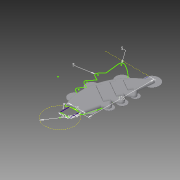
# Autodesk Inventor part: EarWing
Saved by Autodesk Inventor 2014 SP1 (Build 180222100, 222)
## iProperties
Created: 2015-03-17
Part Number: EarWing
Material: Generic
Document SubType Name: Modeling
Designer: Erin
Density: 1 g/cm^3
Appearance: Default
Author: Erin
Autodesk Inventor part; units mm, degrees
ref_plane "YZ Plane" through (0, 0, 0) normal (1, 0, 0) x (0, 1, 0)
ref_plane "XZ Plane" through (0, 0, 0) normal (0, 1, 0) x (-1, 0, 0)
sketch "Sketch1" plane through (0, 0, 0) normal (0, 0, 1) x (1, 0, 0)
  line L0 (-10, -4.740173) -> (10, -4.740173)
  line L1 (10, -4.740173) -> (10, -24.740173)
  line L2 (10, -24.740173) -> (-10, -24.740173)
  line L3 (-10, -24.740173) -> (-10, -4.740173)
  line L4 (-17.5, -4.740173) -> (17.5, -4.740173)
  line L5 (17.5, -4.740173) -> (17.5, 130.259827) construction
  line L6 (17.5, 130.259827) -> (-71.879841, 130.259827) construction
  arc A0 (17.5, -4.740173) -> (-28.622314, 126.472101) centre (-75.017769, 36.45133) ccw
  line L7 (-35.882424, 121.476257) -> (-32.663792, 92.468063)
  line L8 (-32.663792, 92.468063) -> (-40.677059, 83.337371)
  line L9 (-39.242537, 75.611926) -> (-29.283469, 70.385393)
  line L10 (-29.283469, 70.385393) -> (-38.911262, 59.415034)
  line L11 (-37.47674, 51.689589) -> (-26.78782, 46.080029)
  line L12 (-26.78782, 46.080029) -> (-34.350121, 37.463189)
  arc A1 (-28.622314, 126.472101) -> (-35.882424, 121.476257) centre (-30.912921, 122.027653) ccw
  line L13 (-32.915599, 29.737744) -> (-24.548066, 25.346451)
  line L14 (-24.548066, 25.346451) -> (-17.5, -4.740173)
  arc A2 (-40.677059, 83.337371) -> (-39.242537, 75.611926) centre (-36.919057, 80.039278) ccw
  arc A3 (-38.911262, 59.415034) -> (-37.47674, 51.689589) centre (-35.15326, 56.116941) ccw
  arc A4 (-34.350121, 37.463189) -> (-32.915599, 29.737744) centre (-30.592119, 34.165096) ccw
  circle A5 centre (0, -34.740173) radius 30 construction
  arc A6 (15.764218, -8.047675) -> (-16.074353, -8.233283) centre (0, -34.740173) ccw
  line L15 (-17.5, -4.740173) -> (-16.074353, -8.233283)
  line L16 (17.5, -4.740173) -> (15.764218, -8.047675)
  line L17 (-10, -4.740173) -> (10, -4.740173)
  line L18 (10, -4.740173) -> (10, -1.45931)
  line L19 (10, -1.45931) -> (-10, -1.45931)
  line L20 (-10, -1.45931) -> (-10, -4.740173)
  point P0 (0, 0)
  point P1 (0, -4.740173)
  point P2 (-36.857014, 130.259827)
  point P3 (0, -4.740173)
  dimension "d0" = 20
  dimension "d1" = 20
  dimension "d2" = 35
  dimension "d3" = 135
  dimension "d4" = 5
  dimension "d5" = 5
  dimension "d6" = 60
  dimension "d7" = 1
  constraints: 42 end point, 13 point on circle, 9 tangent, 8 parallel, 7 centre point, 6 perpendicular, 2 equal radius, 2 horizontal, 2 midpoint, 2 point on line, 2 vertical alignment, 1 collinear
  measures "d0" distance of L1.end L2.end
  measures "d1" distance of L0.end L1.end
  measures "d2" distance of L4.start L4.end
  measures "d3" distance of L4.end L5.end
  measures "d4" radius of A1
  measures "d5" radius of A2
  measures "d6" diameter of A5
  measures "d7" radial gap between concentric circles of A5 A6
extrude "Extrusion1" add sketch "Sketch1" along normal blind 3 contours L20 L19 L18 L0 A6 | L0 A6 L3 | L3 A6 L15 L4 | L4 L14 L13 A4 L12 L11 A3 L10 L9 A2 L8 L7 A1 A0 L18 L19 L20 | L0 L1 A6 | L4 L16 A6 L1
fillet "Fillet1" radius 5 13 edges at (-33.7473, 126.1467, 3) (-34.2731, 106.9722, 3) (20.5248, 70.0354, 3) (-41.835, 79.1264, 3) (-34.263, 72.9987, 3) (-36.6704, 87.9027, 3) (-40.0692, 55.2041, 3) (-32.1323, 48.8848, 3) (-34.0974, 64.9002, 3) (-35.5081, 33.2523, 3) (-28.7318, 27.5421, 3) (-30.569, 41.7716, 3) (-21.024, 10.3031, 3)
ref_plane "Work Plane1" through (0, 0, 3) normal (0, 0, 1) x (1, 0, 0)
sketch "Sketch2" plane through (0, 0, 3) normal (0, 0, 1) x (1, 0, 0)
  arc A0 (17.5, -4.740173) -> (-28.622314, 126.472101) centre (-75.017769, 36.45133) ccw
  arc A1 (17.5, -4.740173) -> (-28.622314, 126.472101) centre (-75.017769, 36.45133) ccw
  line L0 (-35.882424, 121.476257) -> (-32.663792, 92.468063)
  line L1 (-32.663792, 92.468063) -> (-40.677059, 83.337371)
  arc A2 (-40.677059, 83.337371) -> (-39.242537, 75.611926) centre (-36.919057, 80.039278) ccw
  line L2 (-39.242537, 75.611926) -> (-29.283469, 70.385393)
  line L3 (-29.283469, 70.385393) -> (-38.911262, 59.415034)
  arc A3 (-38.911262, 59.415034) -> (-37.47674, 51.689589) centre (-35.15326, 56.116941) ccw
  line L4 (-37.47674, 51.689589) -> (-26.78782, 46.080029)
  line L5 (-26.78782, 46.080029) -> (-34.350121, 37.463189)
  arc A4 (-34.350121, 37.463189) -> (-32.915599, 29.737744) centre (-30.592119, 34.165096) ccw
  line L6 (-32.915599, 29.737744) -> (-24.548066, 25.346451)
  line L7 (-24.548066, 25.346451) -> (-17.5, -4.740173)
  line L8 (-17.5, -4.740173) -> (-17.5, -4.740173)
  arc A5 (-10, -5.397371) -> (-16.074353, -8.233283) centre (0, -34.740173) ccw
  arc A6 (15.764218, -8.047675) -> (-16.074353, -8.233283) centre (0, -34.740173) ccw
  line L9 (17.5, -4.740173) -> (15.764218, -8.047675)
  line L10 (-28.692137, 88.355038) -> (-5.168136, 101.909269)
  line L11 (-5.168136, 101.909269) -> (-0.503674, 93.813876)
  line L12 (-0.503674, 93.813876) -> (-24.027675, 80.259646)
  line L13 (-24.027675, 80.259646) -> (-28.692137, 88.355038)
  line L14 (-28.000372, 65.795929) -> (5.455455, 85.072752)
  line L15 (5.455455, 85.072752) -> (10.119917, 76.977359)
  line L16 (10.119917, 76.977359) -> (-23.33591, 57.700537)
  line L17 (-23.33591, 57.700537) -> (-28.000372, 65.795929)
  line L18 (-23.904487, 43.113193) -> (13.330015, 64.567241)
  line L19 (13.330015, 64.567241) -> (17.994477, 56.471849)
  line L20 (17.994477, 56.471849) -> (-19.240025, 35.017801)
  line L21 (-19.240025, 35.017801) -> (-23.904487, 43.113193)
  point P0 (0, 0)
  point P1 (-16.074353, -8.233283)
  constraints: 24 end point, 6 parallel, 3 perpendicular, 2 other
extrude "Extrusion3" add sketch "Sketch2" along normal blind 1.5
fillet "Fillet2" radius 5 6 edges at (-26.3599, 84.3073, 4.5) (-25.6681, 61.7482, 4.5) (-21.5723, 39.0655, 4.5) (7.7877, 81.0251, 4.5) (-2.8359, 97.8616, 4.5) (15.6622, 60.5195, 4.5)
sketch "Sketch3" plane through (0, 0, 0) normal (0, 0, 1) x (1, 0, 0)
  circle A0 centre (-30.567755, 123.082332) radius 14.903634
  circle A1 centre (3.412533, 95.957719) radius 12.733671
  circle A2 centre (22.191113, 52.737181) radius 11.866888
  circle A3 centre (20.70075, 16.372315) radius 12.43717
  circle A4 centre (-15.988631, 8.920494) radius 11.808181
  circle A5 centre (-32.356191, 33.660528) radius 8.690238
  circle A6 centre (-37.125354, 56.015978) radius 8.966984
  circle A7 centre (-38.91379, 81.054085) radius 7.772792
  point P0 (0, 0)
  constraints: 8 centre point
extrude "Extrusion4" add sketch "Sketch3" along normal blind 0.3
fillet "Fillet3" radius 3 3 edges at (14.3155, -7.2435, 2.1718) (-14.6001, -7.3935, 2.4057) (-0.3277, -3.7419, 3)
mirror "Mirror1" about plane through (0, 0, 0) normal (1, 0, 0) remove original yes
body "Solid1"
